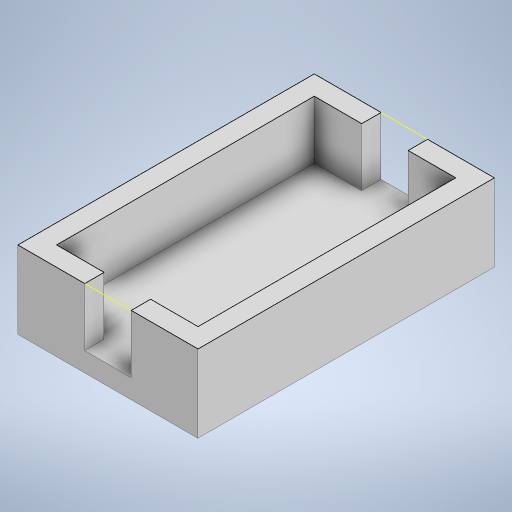
# Autodesk Inventor part: voltage buckboost cover
Saved by Autodesk Inventor 2024 (Build 280153000, 153)
## iProperties
Created: 2024-06-02
Part Number: voltage buckboost cover
Material: Generic
Document SubType Name: Modeling
Designer: ony
Density: 1 g/cm^3
Appearance: Default
Author: ony
Autodesk Inventor part; units mm, degrees
ref_plane "YZ Plane" through (0, 0, 0) normal (1, 0, 0) x (0, 1, 0)
ref_plane "XZ Plane" through (0, 0, 0) normal (0, 1, 0) x (-1, 0, 0)
ref_plane "XY Plane" through (0, 0, 0) normal (0, 0, 1) x (1, 0, 0)
sketch "Sketch1" plane through (0, 0, 0) normal (0, 1, 0) x (-1, 0, 0)
  line L0 (0, 0) -> (36.5, 0)
  line L1 (36.5, 0) -> (36.5, -66.5)
  line L2 (36.5, -66.5) -> (0, -66.5)
  line L3 (0, -66.5) -> (0, 0)
  line L4 (41.5, 5) -> (-5, 5)
  line L5 (-5, 5) -> (-5, -71.5)
  line L6 (-5, -71.5) -> (41.5, -71.5)
  line L7 (41.5, -71.5) -> (41.5, 5)
  line L8 (18.25, 5) -> (24.25, 5)
  line L9 (18.25, -71.5) -> (24.25, -71.5)
  line L10 (24.25, 5) -> (12.25, 5)
  line L11 (12.25, 5) -> (12.25, 0)
  line L12 (12.25, 0) -> (24.25, 0)
  line L13 (24.25, 0) -> (24.25, 5)
  line L14 (24.25, -71.5) -> (12.25, -71.5)
  line L15 (12.25, -71.5) -> (12.25, -66.5)
  line L16 (12.25, -66.5) -> (24.25, -66.5)
  line L17 (24.25, -66.5) -> (24.25, -71.5)
  dimension "d0" = 36.5
  dimension "d1" = 66.5
  dimension "d2" = 5
  dimension "d3" = 6
  dimension "d4" = 6
  dimension "d5" = 12
  dimension "d6" = 12
  constraints: 36 end point, 8 parallel, 4 perpendicular, 4 point on line, 3 horizontal, 2 midpoint, 3 other
  measures "d0" distance of L1.end L2.end
  measures "d1" distance of L0.end L1.end
  measures "d2" distance between parallel lines of L0 L4
  measures "d3" distance of L8.start L8.end
  measures "d4" distance of L9.start L9.end
  measures "d5" distance of L12.end L11.end
  measures "d6" distance of L15.end L16.end
extrude "Extrusion1" add sketch "Sketch1" along normal blind 15 contours L3 L2 L15 L6 L5 L4 L11 L0 | L13 L4 L7 L6 L17 L2 L1 L0
sketch "Sketch2" plane through (0, 0, 0) normal (0, -1, 0) x (1, 0, 0)
  line L0 (-12.25, 5) -> (5, 5) projected
  line L1 (-41.5, -71.5) -> (-41.5, 5) projected
  line L2 (5, 5) -> (-41.5, 5)
  line L3 (-41.5, 5) -> (-41.5, -71.5)
  line L4 (-41.5, -71.5) -> (5, -71.5)
  line L5 (5, -71.5) -> (5, 5)
  point P0 (0, 0)
  constraints: 8 end point, 2 parallel, 1 horizontal, 1 perpendicular
extrude "Extrusion2" add sketch "Sketch2" along normal blind 5
sketch "Sketch3" plane through (0, 15, 0) normal (0, 1, 0) x (1, 0, 0)
  line L0 (5, -5) -> (-41.5, -5) projected
  line L1 (-24.25, -5) -> (-24.25, 0) projected
  line L2 (-41.5, -5) -> (-24.25, -5)
  line L3 (-24.25, -5) -> (-24.25, 0)
  line L4 (-24.25, 0) -> (-36.5, 0) projected
  line L5 (-24.25, 0) -> (-36.5, 0)
  line L6 (-36.5, 0) -> (-36.5, 66.5) projected
  line L7 (-36.5, 0) -> (-36.5, 66.5)
  line L8 (-36.5, 66.5) -> (-24.25, 66.5)
  line L9 (-24.25, 66.5) -> (-24.25, 71.5)
  line L10 (-41.5, 71.5) -> (5, 71.5) projected
  line L11 (-41.5, -5) -> (-41.5, 71.5) projected
  line L12 (-41.5, 71.5) -> (-24.25, 71.5)
  line L13 (-41.5, 71.5) -> (-41.5, -5)
  line L14 (-12.25, 0) -> (-12.25, -5) projected
  line L15 (-12.25, -5) -> (5, -5)
  line L16 (5, -5) -> (5, 71.5) projected
  line L17 (5, -5) -> (5, 71.5)
  line L18 (5, 71.5) -> (-12.25, 71.5)
  line L19 (-12.25, 71.5) -> (-12.25, 66.5) projected
  line L20 (-12.25, 66.5) -> (-12.25, 71.5)
  line L21 (0, 0) -> (-12.25, 0) projected
  line L22 (-12.25, -5) -> (-12.25, 0)
  line L23 (-12.25, 0) -> (0, 0)
  line L24 (0, 66.5) -> (0, 0) projected
  line L25 (0, 0) -> (0, 66.5)
  line L26 (-12.25, 66.5) -> (0, 66.5) projected
  line L27 (0, 66.5) -> (-12.25, 66.5)
  constraints: 32 end point, 10 collinear, 4 perpendicular, 4 point on line
body "Solid1"
